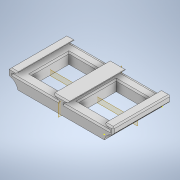
# Autodesk Inventor part: Big well holder 2
Saved by Autodesk Inventor 2021 (Build 250183000, 183)
## iProperties
Created: 2021-05-21
Part Number: Big well holder 2
Material: Generic
Document SubType Name: Modeling
Designer: Olivi
Density: 1 g/cm^3
Appearance: Default
Author: Olivi
Autodesk Inventor part; units mm, degrees
ref_plane "YZ Plane" through (0, 0, 0) normal (1, 0, 0) x (0, 1, 0)
ref_plane "XZ Plane" through (0, 0, 0) normal (0, 1, 0) x (-1, 0, 0)
ref_plane "XY Plane" through (0, 0, 0) normal (0, 0, 1) x (1, 0, 0)
sketch "Sketch1" plane through (0, 0, 0) normal (0, 1, 0) x (-1, 0, 0)
  line L0 (0, 0) -> (0, -85.5)
  line L1 (0, -85.5) -> (127.8, -85.5)
  line L2 (127.8, -85.5) -> (127.8, 0)
  line L3 (127.8, 0) -> (0, 0)
  dimension "d0" = 85.5
  dimension "d1" = 127.8
  constraints: 8 end point, 3 perpendicular, 1 vertical
  measures "d0" distance of L0.start L0.end
  measures "d1" distance of L0.end L1.end
extrude "Extrusion2" add sketch "Sketch1" along normal blind 7
sketch "Sketch3" plane through (0, 7, 0) normal (0, 1, 0) x (1, 0, 0)
  point P0 (0, 0)
sketch "Sketch5" plane through (0, 7, 0) normal (0, 1, 0) x (1, 0, 0)
  line L0 (-127.8, 0) -> (0, 0) projected
  line L1 (-127.8, 0) -> (0, 0)
  line L2 (0, 0) -> (0, 85.5) projected
  line L3 (0, 0) -> (0, 85.5)
  line L4 (0, 85.5) -> (-127.8, 85.5) projected
  line L5 (0, 85.5) -> (-127.8, 85.5)
  line L6 (-127.8, 85.5) -> (-127.8, 0)
  line L7 (-122.8, 80.5) -> (-5, 80.5)
  line L8 (-5, 80.5) -> (-5, 4.1226)
  line L9 (-5, 4.1226) -> (-122.8, 4.1226)
  line L10 (-122.8, 4.1226) -> (-122.8, 80.5)
  line L11 (-127.8, 85.5) -> (-127.8, 0) projected
  dimension "d44" = 5
  dimension "d45" = 5
  dimension "d46" = 5
  constraints: 16 end point, 5 perpendicular, 3 equal length
  measures "d44" distance between parallel lines of L2 L8
  measures "d45" distance between parallel lines of L6 L10
  measures "d46" distance between parallel lines of L4 L7
extrude "Extrusion4" add sketch "Sketch5" along normal blind 10
sketch "Sketch9" plane through (0, 17, 0) normal (0, 1, 0) x (1, 0, 0)
  line L0 (-127.8, 85.5) -> (-127.8, 0) projected
  line L1 (-127.8, 0) -> (-127.8, 85.5)
  line L2 (-127.8, 85.5) -> (0, 85.5)
  line L3 (0, 85.5) -> (0, 0)
  line L4 (0, 0) -> (-127.8, 0)
  line L5 (-122.8, 4.1226) -> (-122.8, 80.5)
  line L6 (-5, 80.5) -> (-5, 4.1226)
  line L7 (-122.8, 80.5) -> (-122.8, 4.1226) projected
  line L8 (-122.8, 15) -> (-5, 15)
  line L9 (-5, 80.5) -> (-5, 4.1226) projected
  line L10 (-122.8, 70.5) -> (-5, 70.5)
  line L11 (-53, 15) -> (-53, 70.5)
  line L12 (-74.8, 70.5) -> (-74.8, 15)
  line L13 (-127.8, 0) -> (0, 0) projected
  line L14 (0, 0) -> (13, 0)
  line L15 (13, 0) -> (13, 85.5)
  line L16 (0, 85.5) -> (-127.8, 85.5) projected
  line L17 (13, 85.5) -> (0, 85.5)
  line L18 (-127.8, 0) -> (-140.8, 0)
  line L19 (-140.8, 0) -> (-140.8, 85.5)
  line L20 (-140.8, 85.5) -> (-127.8, 85.5)
  point P0 (-5, 15)
  dimension "d114" = 15
  dimension "d115" = 15
  dimension "d124" = 48
  dimension "d125" = 48
  dimension "d133" = 13
  dimension "d134" = 13
  constraints: 32 end point, 9 perpendicular, 8 point on line, 2 horizontal, 2 parallel, 1 collinear
  measures "d114" distance between parallel lines of L10 L2
  measures "d115" distance between parallel lines of L4 L8
  measures "d124" distance between parallel lines of L5 L12
  measures "d125" distance between parallel lines of L6 L11
  measures "d133" distance of L13.end L14.end
  measures "d134" distance of L0.end L18.end
ref_plane "Work Plane4" through (-63.9, 0, 0) normal (1, 0, 0) x (0, 0, -1)
ref_plane "Work Plane5" through (-127.8, 0, -42.7) normal (0, 0, 1) x (1, 0, 0)
extrude "Extrusion11" add sketch "Sketch9" along normal blind 5 and the other way blind 5 contours L2 L3 L4 L0 | L0 L18 L19 L20 | L17 L15 L14 L3 | L12 L10 L11 L8
sketch "Sketch26" plane through (0, 0, -85.5) normal (0, 0, -1) x (-1, 0, 0)
  point P0 (0, 0)
sketch "Sketch28" plane through (0, 0, -85.5) normal (0, 0, -1) x (-1, 0, 0)
  point P0 (0, 0)
sketch "Sketch29" plane through (0, 0, -85.5) normal (0, 0, -1) x (-1, 0, 0)
  line L0 (-9, 15.5) -> (-9, 17)
  line L1 (-1, 22) -> (53, 22)
  line L2 (61, 17) -> (61, 15.5)
  line L3 (61, 15.5) -> (-9, 15.5)
  line L4 (66.8, 15.5) -> (66.8, 17)
  line L5 (74.8, 22) -> (128.8, 22)
  line L6 (136.8, 17) -> (136.8, 15.5)
  line L7 (136.8, 15.5) -> (66.8, 15.5)
  line L8 (140.8, 12) -> (140.8, 22) projected
  line L9 (-13, 22) -> (-13, 12) projected
  line L10 (128.8, 22) -> (129.7, 22)
  line L11 (140.8, 22) -> (-13, 22) projected
  line L12 (128.8, 22) -> (128.8, 21.1001)
  line L13 (74.8, 22) -> (74.8, 21.1001)
  line L14 (53, 22) -> (53, 21.1001)
  line L15 (53, 12) -> (53, 22) projected
  line L16 (-1, 22) -> (-1, 21.1001)
  line L17 (74.8, 21.1001) -> (66.8, 17)
  line L18 (53, 21.1001) -> (61, 17)
  line L19 (-1, 21.1001) -> (-9, 17)
  line L20 (128.8, 21.1001) -> (136.8, 17)
  point P0 (0, 0)
  point P1 (145.8, 27)
  point P2 (-18, 27)
  point P3 (0, 27)
  point P4 (127.8, 27)
  dimension "d126" = 1.5
  dimension "d128" = 54
  dimension "d131" = 54
  dimension "d138" = 4
  dimension "d139" = 4
  dimension "d140" = 5.8
  dimension "d182" = 0.9
  constraints: 32 end point, 4 point on line, 2 parallel, 2 perpendicular, 2 vertical, 3 other
  measures "d126" distance of L0.start L0.end
  measures "d128" distance of L1.start L1.end
  measures "d131" distance of L13.start L10.start
  measures "d138" distance from line of L8 L6.start
  measures "d139" distance from line of L9 L0.end
  measures "d140" distance of L4.end L2.start
  measures "d182" distance of L10.start L10.end
extrude "Extrusion13" cut sketch "Sketch29" against normal blind 85.5
sketch "Sketch31" plane through (0, 7, 0) normal (0, 1, 0) x (1, 0, 0)
  line L0 (-5, 70.5) -> (-53, 70.5) projected
  line L1 (-53, 15) -> (-5, 15)
  line L2 (-5, 15) -> (-5, 70.5)
  line L3 (-5, 70.5) -> (-53, 70.5)
  line L4 (-53, 70.5) -> (-53, 15)
  line L5 (-122.8, 80.5) -> (-122.8, 4.1226) projected
  line L6 (-74.8, 70.5) -> (-122.8, 70.5) projected
  line L7 (-122.8, 15) -> (-74.8, 15)
  line L8 (-74.8, 15) -> (-74.8, 70.5)
  line L9 (-74.8, 70.5) -> (-122.8, 70.5)
  line L10 (-122.8, 70.5) -> (-122.8, 15)
  point P0 (0, 0)
  constraints: 16 end point, 4 parallel, 2 horizontal, 2 perpendicular, 2 point on line
extrude "Extrusion15" cut sketch "Sketch31" against normal through all
sketch "Sketch32" plane through (0, 0, 0) normal (0, -1, 0) x (1, 0, 0)
  line L0 (-127.8, -85.5) -> (-127.8, 0) projected
  line L1 (-127.8, 0) -> (0, 0) projected
  line L2 (-127.8, 0) -> (0, 0)
  line L3 (0, 0) -> (0, -85.5) projected
  line L4 (0, 0) -> (0, -85.5)
  line L5 (0, -85.5) -> (-127.8, -85.5)
  line L6 (-136.8, -85.5) -> (-66.8, -85.5) projected
  line L7 (-74.8, -70.5) -> (-122.8, -70.5) projected
  line L8 (-122.8, -15) -> (-74.8, -15)
  line L9 (-74.8, -15) -> (-74.8, -70.5)
  line L10 (-74.8, -70.5) -> (-122.8, -70.5)
  line L11 (-122.8, -70.5) -> (-122.8, -15)
  line L12 (-53, -70.5) -> (-5, -70.5) projected
  line L13 (-53, -15) -> (-5, -15)
  line L14 (-5, -15) -> (-5, -70.5)
  line L15 (-5, -70.5) -> (-53, -70.5)
  line L16 (-53, -70.5) -> (-53, -15)
  point P0 (-74.8, -85.5)
  constraints: 22 end point, 4 parallel, 3 horizontal, 3 perpendicular, 1 point on line
extrude "Extrusion16" add sketch "Sketch32" against normal blind 15
chamfer "Chamfer12" distance 2 angle 45 15 edges at (13, 22, -42.75) (7, 22, -85.5) (7, 22, 0) (-63.9, 22, -85.5) (-63.9, 22, 0) (-140.8, 22, -42.75) (-134.8, 22, -85.5) (-134.8, 22, 0) (-101.8, 15.5, -85.5) (-26, 15.5, -85.5) (-29, 15.5, -70.5) (-5, 15.5, -42.75) (-29, 15.5, -15) (-98.8, 15.5, -15) (-74.8, 15.5, -42.75)
chamfer "Chamfer13" distance 2 angle 45 11 edges at (-53, 15.5, -71.5) (-53, 15.5, -42.75) (-53, 15.5, -14) (-122.8, 15.5, -14) (-122.8, 15.5, -42.75) (-98.8, 15.5, -70.5) (-73.8, 15.5, -70.5) (-101.8, 15.5, 0) (-26, 15.5, 0) (-26, 15.5, -83.5) (-101.8, 15.5, -83.5)
fillet "Fillet2" radius 15 1 edges at (-127.8, 12, -42.75)
fillet "Fillet3" radius 15 1 edges at (0, 12, -42.75)
chamfer "Chamfer15" distance 2 angle 45 3 edges at (13, 12, -42.75) (13, 16, -85.5) (13, 16, 0)
body "Solid2"
